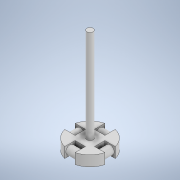
# Autodesk Inventor part: G-6
Saved by Autodesk Inventor 2021 (Build 250183000, 183)
## iProperties
Created: 2021-06-28
Part Number: G-6
Material: Generic
Document SubType Name: Modeling
Designer: Ranjita
Density: 1 g/cm^3
Appearance: Default
Author: Ranjita
Autodesk Inventor part; units mm, degrees
ref_plane "YZ Plane" through (0, 0, 0) normal (1, 0, 0) x (0, 1, 0)
ref_plane "XZ Plane" through (0, 0, 0) normal (0, 1, 0) x (-1, 0, 0)
ref_plane "XY Plane" through (0, 0, 0) normal (0, 0, 1) x (1, 0, 0)
sketch "Sketch1" plane through (0, 0, 0) normal (0, 1, 0) x (-1, 0, 0)
  line L0 (0, 6.665) -> (0, 4.1495) construction
  line L1 (0, 4.1495) -> (0, 0) construction
  line L2 (-1.665, 6.4537) -> (-1.665, 3.1237)
  line L3 (-1.665, 3.1237) -> (1.665, 3.1237)
  line L4 (1.665, 3.1237) -> (1.665, 6.4537)
  line L5 (1.665, 6.4537) -> (-1.665, 3.1237) construction
  line L6 (-1.665, 6.4537) -> (1.665, 3.1237) construction
  line L7 (-6.665, 0) -> (-4.1495, 0) construction
  line L8 (-4.1495, 0) -> (0, 0) construction
  line L9 (-6.4537, -1.665) -> (-3.1237, -1.665)
  line L10 (-3.1237, -1.665) -> (-3.1237, 1.665)
  line L11 (-3.1237, 1.665) -> (-6.4537, 1.665)
  line L12 (-6.4537, 1.665) -> (-3.1237, -1.665) construction
  line L13 (-6.4537, -1.665) -> (-3.1237, 1.665) construction
  line L14 (0, -6.665) -> (0, -4.1495) construction
  line L15 (0, -4.1495) -> (0, 0) construction
  line L16 (1.665, -6.4537) -> (1.665, -3.1237)
  line L17 (1.665, -3.1237) -> (-1.665, -3.1237)
  line L18 (-1.665, -3.1237) -> (-1.665, -6.4537)
  line L19 (-1.665, -6.4537) -> (1.665, -3.1237) construction
  line L20 (1.665, -6.4537) -> (-1.665, -3.1237) construction
  line L21 (6.665, 0) -> (4.1495, 0) construction
  line L22 (4.1495, 0) -> (0, 0) construction
  line L23 (6.4537, 1.665) -> (3.1237, 1.665)
  line L24 (3.1237, 1.665) -> (3.1237, -1.665)
  line L25 (3.1237, -1.665) -> (6.4537, -1.665)
  line L26 (6.4537, -1.665) -> (3.1237, 1.665) construction
  line L27 (6.4537, 1.665) -> (3.1237, -1.665) construction
  arc A0 (-1.665, 6.4537) -> (-6.4537, 1.665) centre (0, 0) ccw
  arc A1 (-6.4537, -1.665) -> (-1.665, -6.4537) centre (0, 0) ccw
  arc A2 (1.665, -6.4537) -> (6.4537, -1.665) centre (0, 0) ccw
  arc A3 (6.4537, 1.665) -> (1.665, 6.4537) centre (0, 0) ccw
  point P0 (0, 4.7887)
  point P1 (-4.7887, 0)
  point P2 (0, -4.7887)
  point P3 (4.7887, 0)
  dimension "d1" = 3.33
  dimension "d4" = 360
  constraints: 56 end point, 8 midpoint, 8 point on circle, 4 centre point, 4 point on line, 1 coincident, 1 collinear, 1 parallel, 1 perpendicular, 1 vertical, 61 other
  measures "d1" distance of L4.end L3.end
extrude "Extrusion1" add sketch "Sketch1" along normal blind 3.33
sketch "Sketch2" plane through (-1.665, 0, 6.4537) normal (1, 0, 0) x (0, 0, -1)
  line L0 (3.33, 0) -> (3.33, 3.33) construction
  line L1 (3.33, 1.665) -> (0, 1.665) construction
  line L2 (0, 0) -> (0, 3.33) construction
  circle A0 centre (1.665, 1.665) radius 1.33
  point P0 (6.4537, 0)
  dimension "d8" = 2.66
  constraints: 3 midpoint, 2 end point, 1 centre point
  measures "d8" diameter of A0
extrude "Extrusion2" add sketch "Sketch2" along normal blind 3.33
pattern_circular "Circular Pattern1" count 4 over 360 about axis through (0, 0, 0) along (0, 1, 0) of "Extrusion2"
sketch "Sketch3" plane through (0, 3.33, 0) normal (0, 1, 0) x (1, 0, 0)
  circle A0 centre (0, 0) radius 1
  dimension "d14" = 2
  constraints: 1 centre point, 1 coincident
  measures "d14" diameter of A0
extrude "Extrusion3" add sketch "Sketch3" along normal blind 30
body "Solid1"
